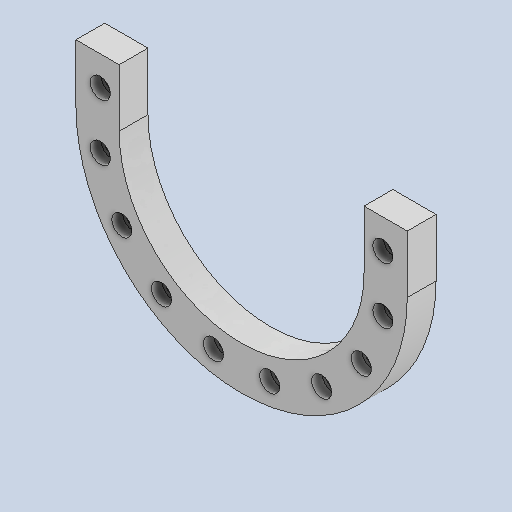
# Autodesk Inventor part: Постель 200
Saved by Autodesk Inventor 2024.2 (Build 282272000, 272)
## iProperties
Created: 2024-04-28
Part Number: Постель 200
Material: Generic
Document SubType Name: Modeling
Designer: admin
Density: 1 g/cm^3
Appearance: Default
Author: pokla
Autodesk Inventor part; units mm, degrees
ref_plane "YZ Plane" through (0, 0, 0) normal (1, 0, 0) x (0, 1, 0)
ref_plane "XZ Plane" through (0, 0, 0) normal (0, 1, 0) x (-1, 0, 0)
ref_plane "XY Plane" through (0, 0, 0) normal (0, 0, 1) x (1, 0, 0)
sketch "Sketch1" plane through (0, 0, 0) normal (0, 0, 1) x (1, 0, 0)
  circle A0 centre (0, 0) radius 200 construction
  line L0 (0, 200) -> (0, 230) construction
  line L1 (0, 200) -> (0, 170) construction
  circle A1 centre (0, 0) radius 170
  circle A2 centre (0, 0) radius 230
  line L2 (-170, 0) -> (-170, 80)
  line L3 (-170, 80) -> (-230, 80)
  line L4 (-230, 80) -> (-230, 0)
  line L5 (170, 0) -> (170, 80)
  line L6 (170, 80) -> (230, 80)
  line L7 (230, 80) -> (230, 0)
  dimension "d13" = 400
  dimension "d26" = 80
  dimension "d36" = 60
  constraints: 16 end point, 6 point on circle, 4 tangent, 4 vertical, 3 coincident, 3 perpendicular, 2 centre point, 2 equal length, 1 horizontal, 1 line through centre, 1 vertical alignment, 2 other
  measures "d26" distance of L2.start L2.end
  measures "d36" distance of L1.end L0.end
extrude "Extrusion1" add sketch "Sketch1" against normal blind 40 contours L5 L6 A2 L3 L2 A1 | L6 L7 A2 | A2 L4 L3 picked at (-188.7937, 40.2131)
sketch "Sketch4" plane through (0, 0, 0) normal (0, 0, 1) x (1, 0, 0)
  circle A0 centre (39.0181, -196.1571) radius 9
  line L0 (0, 0) -> (39.0181, -196.1571) construction
  line L1 (0, 0) -> (0, -276.8337) construction
  dimension "d17" = 18
  dimension "d27" = 200
  dimension "d35" = 11.25
  constraints: 4 end point, 1 centre point, 1 vertical
  measures "d17" diameter of A0
  measures "d27" distance of L0.end L0.start
  measures "d35" angle of L1 L0
extrude "Extrusion4" cut sketch "Sketch4" against normal through all
sketch "Sketch5" plane through (0, 0, 0) normal (0, 0, 1) x (1, 0, 0)
  circle A0 centre (39.0181, -196.1571) radius 9 projected
  circle A1 centre (39.0181, -196.1571) radius 14
  point P0 (0, 0)
  dimension "d23" = 28
  constraints: 1 centre point, 1 coincident
  measures "d23" diameter of A1
extrude "Extrusion5" cut sketch "Sketch5" against normal blind 15
pattern_circular "Circular Pattern3" count 10 over 202.5 about axis through (0, 0, 0) along (0, 0, -1) of "Extrusion4", "Extrusion5" both ways yes
equation "\"d13\" = Шпил_пласт_диам_центров"
equation "\"d27\" = 0.5 * Шпил_пласт_диам_центров"
equation "\"Шпил_пласт_диам_центров\" = 400"
body "Solid1"
